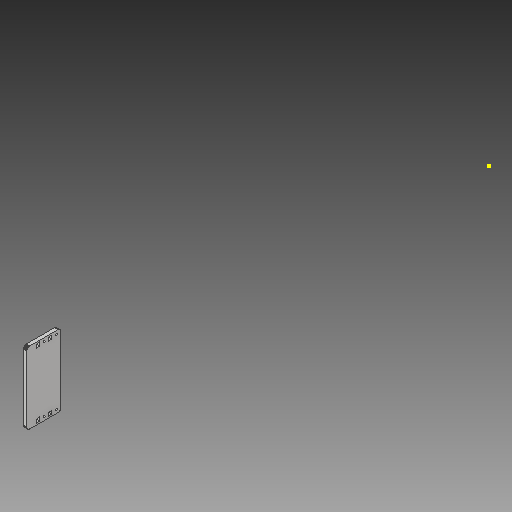
# Autodesk Inventor part: X Axis Brace
Saved by Autodesk Inventor 2018 (Build 220112000, 112)
## iProperties
Created: 2016-07-22
Part Number: X Axis Brace
Material: Generic
Document SubType Name: Modeling
Designer: User
Density: 1 g/cm^3
Appearance: Default
Author: User
Autodesk Inventor part; units mm, degrees
ref_plane "YZ Plane" through (0, 0, 0) normal (1, 0, 0) x (0, 1, 0)
ref_plane "XZ Plane" through (0, 0, 0) normal (0, 1, 0) x (-1, 0, 0)
ref_plane "XY Plane" through (0, 0, 0) normal (0, 0, 1) x (1, 0, 0)
sketch "Sketch1" plane through (0, 0, 0) normal (1, 0, 0) x (0, 1, 0)
  line L0 (122.993, 745.9286) -> (122.843, 746.3036)
  line L1 (122.843, 746.3036) -> (122.593, 746.6537)
  line L2 (122.593, 746.6537) -> (122.268, 746.9036)
  line L3 (122.268, 746.9036) -> (121.868, 747.0536)
  line L4 (121.868, 747.0536) -> (121.4679, 747.1035)
  line L5 (121.4679, 747.1035) -> (121.043, 747.0536)
  line L6 (121.043, 747.0536) -> (120.6679, 746.9036)
  line L7 (120.6679, 746.9036) -> (120.318, 746.6536)
  line L8 (120.318, 746.6536) -> (120.0679, 746.3036)
  line L9 (120.0679, 746.3036) -> (119.9179, 745.9286)
  line L10 (119.9179, 745.9286) -> (119.8679, 745.5036)
  line L11 (119.8679, 745.5036) -> (119.9179, 745.1036)
  line L12 (119.9179, 745.1036) -> (120.068, 744.7035)
  line L13 (120.068, 744.7035) -> (120.3179, 744.3785)
  line L14 (120.3179, 744.3785) -> (120.6679, 744.1285)
  line L15 (120.6679, 744.1285) -> (121.043, 743.9536)
  line L16 (121.043, 743.9536) -> (121.4679, 743.9036)
  line L17 (121.4679, 743.9036) -> (121.868, 743.9536)
  line L18 (121.868, 743.9536) -> (122.268, 744.1285)
  line L19 (122.268, 744.1285) -> (122.593, 744.3785)
  line L20 (122.593, 744.3785) -> (122.8429, 744.7036)
  line L21 (122.8429, 744.7036) -> (122.993, 745.1036)
  line L22 (122.993, 745.1036) -> (123.0681, 745.5035)
  line L23 (123.0681, 745.5035) -> (122.993, 745.9286)
  line L24 (118.518, 759.2036) -> (118.518, 753.2036)
  line L25 (118.518, 753.2036) -> (124.468, 753.2036)
  line L26 (124.468, 753.2036) -> (124.468, 759.2036)
  line L27 (124.468, 759.2036) -> (118.518, 759.2036)
  line L28 (122.9931, 766.9281) -> (122.8431, 767.3031)
  line L29 (122.8431, 767.3031) -> (122.5931, 767.6532)
  line L30 (122.5931, 767.6532) -> (122.268, 767.9031)
  line L31 (122.268, 767.9031) -> (121.868, 768.0531)
  line L32 (121.868, 768.0531) -> (121.468, 768.1034)
  line L33 (121.468, 768.1034) -> (121.0431, 768.0534)
  line L34 (121.0431, 768.0534) -> (120.668, 767.9035)
  line L35 (120.668, 767.9035) -> (120.318, 767.6536)
  line L36 (120.318, 767.6536) -> (120.068, 767.3036)
  line L37 (120.068, 767.3036) -> (119.918, 766.9286)
  line L38 (119.918, 766.9286) -> (119.868, 766.5036)
  line L39 (119.868, 766.5036) -> (119.918, 766.1036)
  line L40 (119.918, 766.1036) -> (120.068, 765.7036)
  line L41 (120.068, 765.7036) -> (120.318, 765.3786)
  line L42 (120.318, 765.3786) -> (120.6679, 765.1286)
  line L43 (120.6679, 765.1286) -> (121.0429, 764.9535)
  line L44 (121.0429, 764.9535) -> (121.4679, 764.9035)
  line L45 (121.4679, 764.9035) -> (121.8679, 764.9534)
  line L46 (121.8679, 764.9534) -> (122.268, 765.1283)
  line L47 (122.268, 765.1283) -> (122.593, 765.3784)
  line L48 (122.593, 765.3784) -> (122.843, 765.7034)
  line L49 (122.843, 765.7034) -> (122.993, 766.1034)
  line L50 (122.993, 766.1034) -> (123.0681, 766.5034)
  line L51 (123.0681, 766.5034) -> (122.9931, 766.9281)
  line L52 (118.518, 780.1036) -> (118.518, 774.1036)
  line L53 (118.518, 774.1036) -> (124.468, 774.1036)
  line L54 (124.468, 774.1036) -> (124.468, 780.1036)
  line L55 (124.468, 780.1036) -> (118.518, 780.1036)
  line L56 (6.468, 780.1036) -> (6.468, 774.1036)
  line L57 (6.468, 774.1036) -> (12.418, 774.1036)
  line L58 (12.418, 774.1036) -> (12.418, 780.1036)
  line L59 (12.418, 780.1036) -> (6.468, 780.1036)
  line L60 (10.9932, 766.9281) -> (10.8431, 767.3031)
  line L61 (10.8431, 767.3031) -> (10.5932, 767.6532)
  line L62 (10.5932, 767.6532) -> (10.2681, 767.9031)
  line L63 (10.2681, 767.9031) -> (9.8681, 768.0531)
  line L64 (9.8681, 768.0531) -> (9.4681, 768.1034)
  line L65 (9.4681, 768.1034) -> (9.0431, 768.0534)
  line L66 (9.0431, 768.0534) -> (8.668, 767.9035)
  line L67 (8.668, 767.9035) -> (8.318, 767.6536)
  line L68 (8.318, 767.6536) -> (8.068, 767.3036)
  line L69 (8.068, 767.3036) -> (7.918, 766.9286)
  line L70 (7.918, 766.9286) -> (7.868, 766.5036)
  line L71 (7.868, 766.5036) -> (7.918, 766.1036)
  line L72 (7.918, 766.1036) -> (8.068, 765.7036)
  line L73 (8.068, 765.7036) -> (8.318, 765.3786)
  line L74 (8.318, 765.3786) -> (8.668, 765.1286)
  line L75 (8.668, 765.1286) -> (9.043, 764.9786)
  line L76 (9.043, 764.9786) -> (9.468, 764.9036)
  line L77 (9.468, 764.9036) -> (9.868, 764.9787)
  line L78 (9.868, 764.9787) -> (10.268, 765.1287)
  line L79 (10.268, 765.1287) -> (10.593, 765.3787)
  line L80 (10.593, 765.3787) -> (10.843, 765.7038)
  line L81 (10.843, 765.7038) -> (10.993, 766.1038)
  line L82 (10.993, 766.1038) -> (11.0682, 766.5037)
  line L83 (11.0682, 766.5037) -> (10.9932, 766.9281)
  line L84 (6.468, 759.2036) -> (6.468, 753.2036)
  line L85 (6.468, 753.2036) -> (12.418, 753.2036)
  line L86 (12.418, 753.2036) -> (12.418, 759.2036)
  line L87 (12.418, 759.2036) -> (6.468, 759.2036)
  line L88 (10.993, 745.9287) -> (10.843, 746.3036)
  line L89 (10.843, 746.3036) -> (10.593, 746.6537)
  line L90 (10.593, 746.6537) -> (10.268, 746.9036)
  line L91 (10.268, 746.9036) -> (9.868, 747.0536)
  line L92 (9.868, 747.0536) -> (9.468, 747.1036)
  line L93 (9.468, 747.1036) -> (9.043, 747.0536)
  line L94 (9.043, 747.0536) -> (8.668, 746.9036)
  line L95 (8.668, 746.9036) -> (8.318, 746.6536)
  line L96 (8.318, 746.6536) -> (8.068, 746.3036)
  line L97 (8.068, 746.3036) -> (7.918, 745.9286)
  line L98 (7.918, 745.9286) -> (7.868, 745.5036)
  line L99 (7.868, 745.5036) -> (7.918, 745.1036)
  line L100 (7.918, 745.1036) -> (8.068, 744.7036)
  line L101 (8.068, 744.7036) -> (8.318, 744.3786)
  line L102 (8.318, 744.3786) -> (8.668, 744.1286)
  line L103 (8.668, 744.1286) -> (9.043, 743.9537)
  line L104 (9.043, 743.9537) -> (9.468, 743.9037)
  line L105 (9.468, 743.9037) -> (9.868, 743.9537)
  line L106 (9.868, 743.9537) -> (10.268, 744.1286)
  line L107 (10.268, 744.1286) -> (10.593, 744.3786)
  line L108 (10.593, 744.3786) -> (10.843, 744.7036)
  line L109 (10.843, 744.7036) -> (10.993, 745.1037)
  line L110 (10.993, 745.1037) -> (11.0681, 745.5036)
  line L111 (11.0681, 745.5036) -> (10.993, 745.9287)
  line L112 (127.4179, 792.1534) -> (127.293, 792.8034)
  line L113 (127.293, 792.8034) -> (127.068, 793.4283)
  line L114 (127.068, 793.4283) -> (126.793, 794.0033)
  line L115 (126.793, 794.0033) -> (126.4181, 794.5534)
  line L116 (126.4181, 794.5534) -> (125.9931, 795.0534)
  line L117 (125.9931, 795.0534) -> (125.4931, 795.4784)
  line L118 (125.4931, 795.4784) -> (124.9681, 795.8534)
  line L119 (124.9681, 795.8534) -> (124.3681, 796.1284)
  line L120 (124.3681, 796.1284) -> (123.7431, 796.3534)
  line L121 (123.7431, 796.3534) -> (123.1181, 796.4784)
  line L122 (123.1181, 796.4784) -> (122.4681, 796.5034)
  line L123 (122.4681, 796.5034) -> (8.4681, 796.5034)
  line L124 (8.4681, 796.5034) -> (7.8181, 796.4784)
  line L125 (7.8181, 796.4784) -> (7.1681, 796.3535)
  line L126 (7.1681, 796.3535) -> (6.5431, 796.1285)
  line L127 (6.5431, 796.1285) -> (5.9681, 795.8535)
  line L128 (5.9681, 795.8535) -> (5.418, 795.4785)
  line L129 (5.418, 795.4785) -> (4.918, 795.0536)
  line L130 (4.918, 795.0536) -> (4.493, 794.5536)
  line L131 (4.493, 794.5536) -> (4.118, 794.0036)
  line L132 (4.118, 794.0036) -> (3.843, 793.4286)
  line L133 (3.843, 793.4286) -> (3.618, 792.8036)
  line L134 (3.618, 792.8036) -> (3.493, 792.1536)
  line L135 (3.493, 792.1536) -> (3.468, 791.5036)
  line L136 (3.468, 791.5036) -> (3.468, 742.9037)
  line L137 (3.468, 742.9037) -> (3.493, 742.2536)
  line L138 (3.493, 742.2536) -> (3.618, 741.6286)
  line L139 (3.618, 741.6286) -> (3.843, 741.0036)
  line L140 (3.843, 741.0036) -> (4.118, 740.4036)
  line L141 (4.118, 740.4036) -> (4.493, 739.8786)
  line L142 (4.493, 739.8786) -> (4.918, 739.3785)
  line L143 (4.918, 739.3785) -> (5.4179, 738.9536)
  line L144 (5.4179, 738.9536) -> (5.968, 738.5786)
  line L145 (5.968, 738.5786) -> (6.543, 738.3035)
  line L146 (6.543, 738.3035) -> (7.1679, 738.0785)
  line L147 (7.1679, 738.0785) -> (7.8179, 737.9534)
  line L148 (7.8179, 737.9534) -> (8.4679, 737.9034)
  line L149 (8.4679, 737.9034) -> (122.4679, 737.9034)
  line L150 (122.4679, 737.9034) -> (123.1179, 737.9534)
  line L151 (123.1179, 737.9534) -> (123.7433, 738.0784)
  line L152 (123.7433, 738.0784) -> (124.3683, 738.3034)
  line L153 (124.3683, 738.3034) -> (124.9683, 738.5785)
  line L154 (124.9683, 738.5785) -> (125.4933, 738.9534)
  line L155 (125.4933, 738.9534) -> (125.9933, 739.3784)
  line L156 (125.9933, 739.3784) -> (126.4183, 739.8784)
  line L157 (126.4183, 739.8784) -> (126.7933, 740.4034)
  line L158 (126.7933, 740.4034) -> (127.0683, 741.0034)
  line L159 (127.0683, 741.0034) -> (127.2933, 741.6284)
  line L160 (127.2933, 741.6284) -> (127.4183, 742.2534)
  line L161 (127.4183, 742.2534) -> (127.4678, 742.8973)
  line L162 (127.4678, 742.8973) -> (127.4678, 791.5034)
  line L163 (127.4678, 791.5034) -> (127.4179, 792.1534)
  point P0 (0, 0)
  constraints: 328 end point, 60 parallel, 58 perpendicular, 1 collinear
extrude "Extrusion1" add sketch "Sketch1" along normal blind 6
sketch "Sketch2" plane through (0, 0, 0) normal (-1, 0, 0) x (0, 0, 1)
  line L0 (780.1036, 118.468) -> (780.1036, 124.418) projected
  line L1 (774.1036, 118.468) -> (780.1036, 118.468) projected
  line L2 (774.1036, 124.418) -> (774.1036, 118.468) projected
  line L3 (780.1036, 124.418) -> (774.1036, 124.418) projected
  line L4 (780.1036, 6.418) -> (780.1036, 12.368) projected
  line L5 (774.1036, 6.418) -> (780.1036, 6.418) projected
  line L6 (774.1036, 12.368) -> (774.1036, 6.418) projected
  line L7 (780.1036, 12.368) -> (774.1036, 12.368) projected
  line L8 (759.2036, 118.468) -> (759.2036, 124.418) projected
  line L9 (753.2036, 118.468) -> (759.2036, 118.468) projected
  line L10 (753.2036, 124.418) -> (753.2036, 118.468) projected
  line L11 (759.2036, 124.418) -> (753.2036, 124.418) projected
  line L12 (759.2036, 6.418) -> (759.2036, 12.368) projected
  line L13 (753.2036, 6.418) -> (759.2036, 6.418) projected
  line L14 (753.2036, 12.368) -> (753.2036, 6.418) projected
  line L15 (759.2036, 12.368) -> (753.2036, 12.368) projected
  line L16 (745.9286, 122.943) -> (745.5035, 123.0181) projected
  line L17 (746.3036, 122.793) -> (745.9286, 122.943) projected
  line L18 (746.6537, 122.543) -> (746.3036, 122.793) projected
  line L19 (746.9036, 122.218) -> (746.6537, 122.543) projected
  line L20 (747.0536, 121.818) -> (746.9036, 122.218) projected
  line L21 (747.1035, 121.4179) -> (747.0536, 121.818) projected
  line L22 (747.0536, 120.993) -> (747.1035, 121.4179) projected
  line L23 (746.9036, 120.6179) -> (747.0536, 120.993) projected
  line L24 (746.6536, 120.268) -> (746.9036, 120.6179) projected
  line L25 (746.3036, 120.0179) -> (746.6536, 120.268) projected
  line L26 (745.9286, 119.8679) -> (746.3036, 120.0179) projected
  line L27 (745.5036, 119.8179) -> (745.9286, 119.8679) projected
  line L28 (745.1036, 119.8679) -> (745.5036, 119.8179) projected
  line L29 (744.7035, 120.018) -> (745.1036, 119.8679) projected
  line L30 (744.3785, 120.2679) -> (744.7035, 120.018) projected
  line L31 (744.1285, 120.6179) -> (744.3785, 120.2679) projected
  line L32 (743.9536, 120.993) -> (744.1285, 120.6179) projected
  line L33 (743.9036, 121.4179) -> (743.9536, 120.993) projected
  line L34 (743.9536, 121.818) -> (743.9036, 121.4179) projected
  line L35 (744.1285, 122.218) -> (743.9536, 121.818) projected
  line L36 (744.3785, 122.543) -> (744.1285, 122.218) projected
  line L37 (744.7036, 122.7929) -> (744.3785, 122.543) projected
  line L38 (745.1036, 122.943) -> (744.7036, 122.7929) projected
  line L39 (745.5035, 123.0181) -> (745.1036, 122.943) projected
  line L40 (745.9287, 10.943) -> (745.5036, 11.0182) projected
  line L41 (746.3036, 10.793) -> (745.9287, 10.943) projected
  line L42 (746.6537, 10.543) -> (746.3036, 10.793) projected
  line L43 (746.9036, 10.218) -> (746.6537, 10.543) projected
  line L44 (747.0536, 9.818) -> (746.9036, 10.218) projected
  line L45 (747.1036, 9.418) -> (747.0536, 9.818) projected
  line L46 (747.0536, 8.993) -> (747.1036, 9.418) projected
  line L47 (746.9036, 8.618) -> (747.0536, 8.993) projected
  line L48 (746.6536, 8.268) -> (746.9036, 8.618) projected
  line L49 (746.3036, 8.018) -> (746.6536, 8.268) projected
  line L50 (745.9286, 7.868) -> (746.3036, 8.018) projected
  line L51 (745.5036, 7.818) -> (745.9286, 7.868) projected
  line L52 (745.1036, 7.868) -> (745.5036, 7.818) projected
  line L53 (744.7036, 8.018) -> (745.1036, 7.868) projected
  line L54 (744.3786, 8.268) -> (744.7036, 8.018) projected
  line L55 (744.1286, 8.618) -> (744.3786, 8.268) projected
  line L56 (743.9537, 8.993) -> (744.1286, 8.618) projected
  line L57 (743.9037, 9.418) -> (743.9537, 8.993) projected
  line L58 (743.9537, 9.818) -> (743.9037, 9.418) projected
  line L59 (744.1286, 10.218) -> (743.9537, 9.818) projected
  line L60 (744.3786, 10.543) -> (744.1286, 10.218) projected
  line L61 (744.7036, 10.793) -> (744.3786, 10.543) projected
  line L62 (745.1037, 10.943) -> (744.7036, 10.793) projected
  line L63 (745.5036, 11.0182) -> (745.1037, 10.943) projected
  line L64 (766.9281, 122.9431) -> (766.5034, 123.0181) projected
  line L65 (767.3031, 122.7931) -> (766.9281, 122.9431) projected
  line L66 (767.6532, 122.5431) -> (767.3031, 122.7931) projected
  line L67 (767.9031, 122.218) -> (767.6532, 122.5431) projected
  line L68 (768.0531, 121.818) -> (767.9031, 122.218) projected
  line L69 (768.1034, 121.418) -> (768.0531, 121.818) projected
  line L70 (768.0534, 120.9931) -> (768.1034, 121.418) projected
  line L71 (767.9035, 120.618) -> (768.0534, 120.9931) projected
  line L72 (767.6536, 120.268) -> (767.9035, 120.618) projected
  line L73 (767.3036, 120.018) -> (767.6536, 120.268) projected
  line L74 (766.9286, 119.868) -> (767.3036, 120.018) projected
  line L75 (766.5036, 119.818) -> (766.9286, 119.868) projected
  line L76 (766.1036, 119.868) -> (766.5036, 119.818) projected
  line L77 (765.7036, 120.018) -> (766.1036, 119.868) projected
  line L78 (765.3786, 120.268) -> (765.7036, 120.018) projected
  line L79 (765.1286, 120.618) -> (765.3786, 120.268) projected
  line L80 (764.9535, 120.993) -> (765.1286, 120.618) projected
  line L81 (764.9035, 121.4179) -> (764.9535, 120.993) projected
  line L82 (764.9534, 121.8179) -> (764.9035, 121.4179) projected
  line L83 (765.1283, 122.218) -> (764.9534, 121.8179) projected
  line L84 (765.3784, 122.543) -> (765.1283, 122.218) projected
  line L85 (765.7034, 122.793) -> (765.3784, 122.543) projected
  line L86 (766.1034, 122.943) -> (765.7034, 122.793) projected
  line L87 (766.5034, 123.0181) -> (766.1034, 122.943) projected
  line L88 (766.9281, 10.9432) -> (766.5037, 11.0182) projected
  line L89 (767.3031, 10.7931) -> (766.9281, 10.9432) projected
  line L90 (767.6532, 10.5432) -> (767.3031, 10.7931) projected
  line L91 (767.9031, 10.2181) -> (767.6532, 10.5432) projected
  line L92 (768.0531, 9.8181) -> (767.9031, 10.2181) projected
  line L93 (768.1034, 9.4181) -> (768.0531, 9.8181) projected
  line L94 (768.0534, 8.9931) -> (768.1034, 9.4181) projected
  line L95 (767.9035, 8.618) -> (768.0534, 8.9931) projected
  line L96 (767.6536, 8.268) -> (767.9035, 8.618) projected
  line L97 (767.3036, 8.018) -> (767.6536, 8.268) projected
  line L98 (766.9286, 7.868) -> (767.3036, 8.018) projected
  line L99 (766.5036, 7.818) -> (766.9286, 7.868) projected
  line L100 (766.1036, 7.868) -> (766.5036, 7.818) projected
  line L101 (765.7036, 8.018) -> (766.1036, 7.868) projected
  line L102 (765.3786, 8.268) -> (765.7036, 8.018) projected
  line L103 (765.1286, 8.618) -> (765.3786, 8.268) projected
  line L104 (764.9786, 8.993) -> (765.1286, 8.618) projected
  line L105 (764.9036, 9.418) -> (764.9786, 8.993) projected
  line L106 (764.9787, 9.818) -> (764.9036, 9.418) projected
  line L107 (765.1287, 10.218) -> (764.9787, 9.818) projected
  line L108 (765.3787, 10.543) -> (765.1287, 10.218) projected
  line L109 (765.7038, 10.793) -> (765.3787, 10.543) projected
  line L110 (766.1038, 10.943) -> (765.7038, 10.793) projected
  line L111 (766.5037, 11.0182) -> (766.1038, 10.943) projected
  line L112 (792.1534, 127.3679) -> (792.8034, 127.243) projected
  line L113 (791.5034, 127.4179) -> (792.1534, 127.3679) projected
  line L114 (742.8973, 127.4179) -> (791.5034, 127.4179) projected
  line L115 (742.2534, 127.3683) -> (742.8973, 127.4179) projected
  line L116 (741.6284, 127.2434) -> (742.2534, 127.3683) projected
  line L117 (741.0034, 127.0183) -> (741.6284, 127.2434) projected
  line L118 (740.4034, 126.7433) -> (741.0034, 127.0183) projected
  line L119 (739.8784, 126.3683) -> (740.4034, 126.7433) projected
  line L120 (739.3784, 125.9433) -> (739.8784, 126.3683) projected
  line L121 (738.9534, 125.4433) -> (739.3784, 125.9433) projected
  line L122 (738.5785, 124.9183) -> (738.9534, 125.4433) projected
  line L123 (738.3034, 124.3183) -> (738.5785, 124.9183) projected
  line L124 (738.0784, 123.6933) -> (738.3034, 124.3183) projected
  line L125 (737.9534, 123.0679) -> (738.0784, 123.6933) projected
  line L126 (737.9034, 122.4179) -> (737.9534, 123.0679) projected
  line L127 (737.9034, 8.4179) -> (737.9034, 122.4179) projected
  line L128 (737.9534, 7.7679) -> (737.9034, 8.4179) projected
  line L129 (738.0785, 7.1179) -> (737.9534, 7.7679) projected
  line L130 (738.3035, 6.493) -> (738.0785, 7.1179) projected
  line L131 (738.5786, 5.918) -> (738.3035, 6.493) projected
  line L132 (738.9536, 5.368) -> (738.5786, 5.918) projected
  line L133 (739.3785, 4.868) -> (738.9536, 5.368) projected
  line L134 (739.8786, 4.443) -> (739.3785, 4.868) projected
  line L135 (740.4036, 4.068) -> (739.8786, 4.443) projected
  line L136 (741.0036, 3.793) -> (740.4036, 4.068) projected
  line L137 (741.6286, 3.568) -> (741.0036, 3.793) projected
  line L138 (742.2536, 3.443) -> (741.6286, 3.568) projected
  line L139 (742.9037, 3.418) -> (742.2536, 3.443) projected
  line L140 (791.5036, 3.418) -> (742.9037, 3.418) projected
  line L141 (792.1536, 3.443) -> (791.5036, 3.418) projected
  line L142 (792.8036, 3.568) -> (792.1536, 3.443) projected
  line L143 (793.4286, 3.793) -> (792.8036, 3.568) projected
  line L144 (794.0036, 4.068) -> (793.4286, 3.793) projected
  line L145 (794.5536, 4.443) -> (794.0036, 4.068) projected
  line L146 (795.0536, 4.868) -> (794.5536, 4.443) projected
  line L147 (795.4785, 5.368) -> (795.0536, 4.868) projected
  line L148 (795.8535, 5.9181) -> (795.4785, 5.368) projected
  line L149 (796.1285, 6.4931) -> (795.8535, 5.9181) projected
  line L150 (796.3535, 7.1181) -> (796.1285, 6.4931) projected
  line L151 (796.4784, 7.7681) -> (796.3535, 7.1181) projected
  line L152 (796.5034, 8.4181) -> (796.4784, 7.7681) projected
  line L153 (796.5034, 122.4181) -> (796.5034, 8.4181) projected
  line L154 (796.4784, 123.0681) -> (796.5034, 122.4181) projected
  line L155 (796.3534, 123.6931) -> (796.4784, 123.0681) projected
  line L156 (796.1284, 124.3181) -> (796.3534, 123.6931) projected
  line L157 (795.8534, 124.9181) -> (796.1284, 124.3181) projected
  line L158 (795.4784, 125.4431) -> (795.8534, 124.9181) projected
  line L159 (795.0534, 125.9431) -> (795.4784, 125.4431) projected
  line L160 (794.5534, 126.3681) -> (795.0534, 125.9431) projected
  line L161 (794.0033, 126.743) -> (794.5534, 126.3681) projected
  line L162 (793.4283, 127.018) -> (794.0033, 126.743) projected
  line L163 (792.8034, 127.243) -> (793.4283, 127.018) projected
  line L164 (745.5036, 119.8679) -> (745.9286, 119.9179) projected
  line L165 (745.5035, 123.0181) -> (745.5036, 119.8679)
  line L166 (766.5034, 123.0181) -> (766.5036, 119.818)
  line L167 (745.5036, 11.0182) -> (745.5036, 7.818)
  line L168 (766.5037, 11.0182) -> (766.5036, 7.818)
  point P0 (0, 0)
  point P1 (745.5036, 121.443)
  point P2 (766.5035, 121.4181)
  point P3 (745.5036, 9.4181)
  point P4 (766.5037, 9.4181)
  constraints: 8 end point, 4 midpoint, 1 other
hole "Hole1" at (0, 121.443, 745.5036) at (0, 121.4181, 766.5035) at (0, 9.4181, 745.5036) at (0, 9.4181, 766.5037) direction (1, 0, 0) diameter 3.2 end through all
sketch "Sketch3" plane through (6, 0, 0) normal (1, 0, 0) x (0, 0, -1)
  point P0 (0, 0)
body "Solid1"
